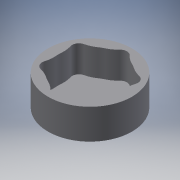
# Autodesk Inventor part: embrague_1
Saved by Autodesk Inventor 2018 (Build 220112000, 112)
## iProperties
Created: 2018-08-07
Part Number: embrague_1
Material: Generic
Document SubType Name: Sheet Metal
Designer: Bardo91
Density: 1 g/cm^3
Sheet Metal Rule: Default_mm
Appearance: Default
Author: Bardo91
Autodesk Inventor part; units mm, degrees
ref_plane "YZ Plane" through (0, 0, 0) normal (1, 0, 0) x (0, 1, 0)
ref_plane "XZ Plane" through (0, 0, 0) normal (0, 1, 0) x (-1, 0, 0)
ref_plane "XY Plane" through (0, 0, 0) normal (0, 0, 1) x (1, 0, 0)
sketch "Sketch6" plane through (0, 0, 0) normal (0, 0, 1) x (1, 0, 0)
  circle A0 centre (0, 0) radius 12.5
  dimension "d29" = 25
  constraints: 1 centre point, 1 coincident
  measures "d29" diameter of A0
extrude "base" add sketch "Sketch6" along normal blind 9
sketch "Sketch8" plane through (0, 0, 9) normal (0, 0, 1) x (1, 0, 0)
  circle A0 centre (0, 0) radius 9.4
  dimension "d39" = 18.8
  constraints: 1 centre point, 1 coincident
  measures "d39" diameter of A0
extrude "Extrusion8" cut sketch "Sketch8" against normal blind 8
sketch "Sketch7" plane through (0, 0, 9) normal (0, 0, 1) x (1, 0, 0)
  line L0 (0, 0) -> (0, 9)
  circle A0 centre (0, 9) radius 2
  dimension "d33" = 9
  dimension "d34" = 4
  constraints: 2 end point, 1 centre point, 1 coincident, 1 vertical
  measures "d33" distance of L0.start L0.end
  measures "d34" diameter of A0
extrude "ball_place" cut sketch "Sketch7" against normal blind 8
fillet "Fillet5" radius 8 2 edges at (-1.9913, 9.1867, 5) (1.9913, 9.1867, 5)
pattern_circular "Circular Pattern2" count 6 over 360 about axis through (0, 0, 9) along (0, 0, -1) of "ball_place", "Fillet5"
equation "\"BendRadius\" = Thickness"
equation "\"BendReliefWidth\" = Thickness"
equation "\"BendReliefDepth\" = 0.5 * Thickness"
equation "\"CornerReliefSize\" = 4 * Thickness"
equation "\"MinimumRemnant\" = 2 * Thickness"
equation "\"TransitionRadius\" = BendRadius"
equation "\"JacobiRadiusSize\" = BendRadius"
equation "\"GapSize\" = Thickness"
equation "\"Thickness\" = 0.5"
body "Solid2"
